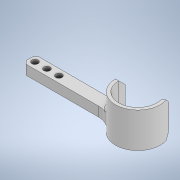
# Autodesk Inventor part: squirrely_leg_front
Saved by Autodesk Inventor 2020 (Build 240168000, 168)
## iProperties
Created: 2019-05-01
Part Number: squirrely_leg_front
Material: Generic
Document SubType Name: Modeling
Designer: mfans
Density: 1 g/cm^3
Appearance: Default
Author: mfans
Autodesk Inventor part; units mm, degrees
note: some values were not read from the file. Chosen so that the rebuilt part matches the saved one: edges of "Fillet1".
ref_plane "YZ Plane" through (0, 0, 0) normal (1, 0, 0) x (0, 1, 0)
ref_plane "XZ Plane" through (0, 0, 0) normal (0, 1, 0) x (-1, 0, 0)
ref_plane "XY Plane" through (0, 0, 0) normal (0, 0, 1) x (1, 0, 0)
sketch "Sketch1" plane through (0, 0, 0) normal (0, 1, 0) x (-1, 0, 0)
  line L0 (28, 4) -> (-28, 4)
  line L1 (-28, 4) -> (-28, -4)
  line L2 (-28, -4) -> (28, -4)
  line L3 (28, -4) -> (28, 4)
  line L4 (28, 4) -> (-28, -4) construction
  line L5 (-28, 4) -> (28, -4) construction
  point P0 (0, 0)
  dimension "d0" = 8
  dimension "d1" = 56
  constraints: 12 end point, 2 midpoint, 2 parallel, 1 horizontal, 1 perpendicular
  measures "d0" distance between parallel lines of L0 L2
  measures "d1" distance of L1.end L2.end
extrude "Extrusion1" add sketch "Sketch1" along normal blind 6
sketch "Sketch2" plane through (0, 6, 0) normal (0, 1, 0) x (1, 0, 0)
  line L0 (28, -4) -> (28, 4) projected
  line L1 (28, 4) -> (-28, 4) projected
  line L2 (-28, 4) -> (-28, -4) projected
  line L3 (-28, -4) -> (28, -4) projected
  point P0 (0, 0)
  point P1 (-17, 0)
  point P2 (-24.5, 0)
  point P3 (-9.5, 0)
  dimension "d4" = 7.5
  dimension "d5" = 11
  dimension "d14" = 7.5
  measures "d4" distance of point (-24.5, 0) point (-17, 0)
  measures "d5" distance from line of L2 point (-17, 0)
  measures "d14" distance of point (-17, 0) point (-9.5, 0)
hole "Hole1" at (-17, 6, 0) at (-24.5, 6, 0) at (-9.5, 6, 0) direction (0, -1, 0) diameter 4 end through all
sketch "Sketch3" plane through (0, 6, 0) normal (0, 1, 0) x (1, 0, 0)
  line L0 (28, -4) -> (28, 4) projected
  arc A0 (28, 0) -> (49.7378, 7.0126) centre (40, 0) ccw
  arc A1 (26, 0) -> (51.4773, 8.0169) centre (40, 0) ccw
  line L1 (51.4773, 8.0169) -> (49.7378, 7.0126)
  line L2 (28, 0) -> (28, 4)
  line L3 (28, 4) -> (-28, 4) projected
  line L4 (26, 4) -> (26, 0)
  point P0 (0, 0)
  dimension "d15" = 2
  dimension "d16" = 0
  dimension "d17" = 60
  dimension "d22" = 12
  constraints: 6 end point, 4 point on circle, 3 tangent, 2 centre point, 1 coincident, 1 collinear, 1 midpoint, 1 point on line
  measures "d15" radial gap between concentric circles of A1 A0
  measures "d16" vertical distance of point (0, 0) A0.centre
  measures "d17" angle of L0 L1
  measures "d22" radius of A0
extrude "Extrusion2" add sketch "Sketch3" along normal blind 16 and the other way blind 6
chamfer "Chamfer1" distance 5 angle 45 2 edges at (26, 6, -2) (26.1467, 6, 2.0212)
chamfer "Chamfer2" distance 2 angle 45 2 edges at (-28, 3, 4) (-28, 3, -4)
chamfer "Chamfer3" distance 4 angle 45 3 edges at (27, 22, -4) (50.6076, 22, -7.5147) (50.6076, 0, -7.5147)
fillet "Fillet1" radius 12 1 edges at (26.5836, 3, 4)
fillet "Fillet2" radius 4 1 edges at (24.865, 8.9761, 5.2631)
body "Solid1"
